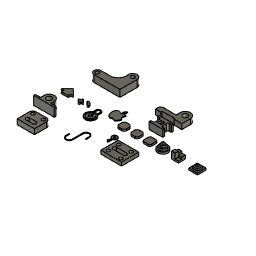
4~10 v4 (Autodesk Fusion 360 design; units mm, degrees)
Autodesk Fusion 360 part; units mm, degrees
note: some values were not read from the file. Set by a fixed rule: which sketch regions a step uses.
sketch "스케치1" plane through (0, 0, 0) normal (0, 0, 1) x (1, 0, 0)
  line L0 (-16, 16) -> (16, 16)
  line L1 (16, 16) -> (16, -16)
  line L2 (16, -16) -> (-16, -16)
  line L3 (-16, -16) -> (-16, 16)
  line L4 (-16, 16) -> (16, -16) construction
  line L5 (16, 16) -> (-16, -16) construction
  circle A0 centre (-16, 16) radius 17
  line L6 (-13, 13) -> (13, 13)
  line L7 (13, 13) -> (13, -13)
  line L8 (13, -13) -> (-13, -13)
  line L9 (-13, -13) -> (-13, 13)
  line L10 (-13, 13) -> (13, -13) construction
  line L11 (13, 13) -> (-13, -13) construction
  circle A1 centre (-13, -13) radius 12
  arc A2 (-32.6238, 19.5565) -> (-22.3496, -20.5223) centre (16.6071, 10.8206) ccw
  circle A3 centre (13, -13) radius 12
  circle A4 centre (0, -30.7482) radius 10
  circle A5 centre (16, 16) radius 17
  circle A6 centre (0, 37.7486) radius 10
  arc A7 (23.2744, -19.1998) -> (32.5898, 19.7118) centre (-16.632, 10.9247) ccw
  circle A8 centre (40, 16) radius 18
  arc A9 (-5.9259, 29.6935) -> (5.9259, 29.6935) centre (0, 37.7486) ccw
  arc A10 (5.9091, -22.6809) -> (-5.9091, -22.6809) centre (0, -30.7482) ccw
  dimension "d1" = 32
  dimension "d2" = 32
  dimension "d3" = 34
  dimension "d4" = 26
  dimension "d5" = 26
  dimension "d6" = 24
  dimension "d7" = 50
  dimension "d9" = 24
  dimension "d14" = 20
  dimension "d15" = 34
  dimension "d16" = 20
  dimension "d17" = 50
  dimension "d18" = 36
  dimension "d19" = 24
  dimension "d20" = 32
  constraint horizontal L0
  constraint perpendicular L0 L1
  constraint parallel L0 L2
  constraint parallel L1 L3
  constraint coincident L4 origin
  constraint coincident L5 origin
  constraint coincident L0.start L3.end
  constraint horizontal L6
  constraint perpendicular L6 L7
  constraint parallel L6 L8
  constraint parallel L7 L9
  constraint coincident L10 origin
  constraint coincident L11 origin
  constraint coincident L8.end L9.start
  constraint tangent A1 A2
  constraint coincident A1 A2.end
  constraint coincident A0 A2.start
  constraint coincident L7.end L8.start
  constraint tangent A3 A4
  constraint tangent A1 A4
  constraint coincident L0.end L1.start
  constraint tangent A0 A6
  constraint tangent A5 A6
  constraint coincident A3 A7.start
  constraint coincident A5 A7.end
  constraint tangent A5 A9
  constraint tangent A0 A9
  constraint coincident A6 A9.end
  constraint coincident A5 A9.end
  constraint coincident A0 A9.start
  constraint tangent A1 A10
  constraint coincident A3 A10.start
  constraint coincident A4 A10.start
  constraint coincident A1 A10.end
  constraint coincident A4 A10.end
  measures "d1" distance of L1.end L2.end
  measures "d2" distance of L0.end L1.end
  measures "d3" diameter of A0
  measures "d4" distance of L7.end L8.end
  measures "d5" distance of L6.end L7.end
  measures "d6" diameter of A1
  measures "d7" radius of A2
  measures "d9" diameter of A3
  measures "d14" diameter of A4
  measures "d15" diameter of A5
  measures "d16" diameter of A6
  measures "d17" radius of A7
  measures "d18" diameter of A8
  measures "d19" distance of L1 A8.centre
  measures "d20" distance of L2 A8.centre
extrude "돌출1" add sketch "스케치1" along normal blind 4 contours L0 L1 A0 A5 A8 | L0 A0 L6 A5 | L0 A0 A5 | L0 L1 A0 L6 L7 A5 | L0 L3 A0 L6 L9 A5 | L0 L3 A0 A2 A5 | A0 A5 A6 A9 | A0 L6 L7 A5 | A0 L6 A5 | L1 A3 A5 A7 A8 | L1 L7 A3 A5 | A0 L6 L9 A5 | A0 L7 L8 L9 A1 A3 A5 | L1 L2 A3 | L1 L2 L7 L8 A3 | L3 A0 L9 A1 | L3 A0 A1 A2 | L7 L8 A3 | L2 L3 L8 L9 A1 | L2 L3 A1 | L8 L9 A1 | L2 A1 A3 A4 A10 | L2 L8 A1 A3 makes body 1
sketch "스케치2" plane through (0, 0, 0) normal (0, 0, 1) x (1, 0, 0)
  arc A0 (-5.9259, 29.6935) -> (-32.6238, 19.5565) centre (-16, 16) ccw
  arc A1 (27.2708, 28.7267) -> (5.9259, 29.6935) centre (16, 16) ccw
  arc A2 (-5.9259, 29.6935) -> (5.9259, 29.6935) centre (0, 37.7486) ccw
  arc A3 (0, 33.006) -> (12.0073, 53.7864) centre (-6.1442, 50.4155) ccw
  arc A4 (12.0073, 53.7864) -> (0, 33.006) centre (21.5511, 34.4126) ccw
  line L0 (-16, 33) -> (16, 33)
  dimension "d24" = 24
  dimension "d35" = 16
  constraint coincident A0 L0.start
  constraint coincident A1 L0.end
  constraint tangent A1 L0
  constraint horizontal L0
  measures "d24" distance of A3.end A3.start
  measures "d35" horizontal distance of A3.start L0.start
extrude "돌출2" add sketch "스케치2" along normal blind 4 separate body contours A3 A4 makes body 2
move_body "이동1" bodies 1 2 to x (1, 0, 0) y (0, 0, 1) z (0, -1, 0) at (0, 37.7486, 22.2514)
sketch "스케치3" plane through (0, 0, 0) normal (0, 0, 1) x (1, 0, 0)
  line L0 (67.5, 22.5) -> (82.5, 22.5)
  line L1 (97.5, 7.5) -> (97.5, -7.5)
  line L2 (82.5, -22.5) -> (67.5, -22.5)
  line L3 (52.5, -7.5) -> (52.5, 7.5)
  line L4 (52.5, 22.5) -> (97.5, -22.5) construction
  line L5 (97.5, 22.5) -> (52.5, -22.5) construction
  arc A0 (67.5, 22.5) -> (52.5, 7.5) centre (67.5, 7.5) ccw
  arc A1 (97.5, 7.5) -> (82.5, 22.5) centre (82.5, 7.5) ccw
  arc A2 (52.5, -7.5) -> (67.5, -22.5) centre (67.5, -7.5) ccw
  arc A3 (82.5, -22.5) -> (97.5, -7.5) centre (82.5, -7.5) ccw
  line L6 (137.5, 22.5) -> (162.5, 22.5)
  line L7 (172.5, 12.5) -> (172.5, -12.5)
  line L8 (162.5, -22.5) -> (137.5, -22.5)
  line L9 (127.5, -12.5) -> (127.5, 12.5)
  line L10 (127.5, 22.5) -> (172.5, -22.5) construction
  line L11 (172.5, 22.5) -> (127.5, -22.5) construction
  line L12 (137.5, 22.5) -> (127.5, 12.5)
  line L13 (162.5, 22.5) -> (172.5, 12.5)
  line L14 (127.5, -12.5) -> (137.5, -22.5)
  line L15 (172.5, -12.5) -> (162.5, -22.5)
  line L16 (207.5, 22.5) -> (237.5, 22.5)
  line L17 (247.5, 17.5) -> (247.5, -12.5)
  line L18 (242.5, -22.5) -> (212.5, -22.5)
  line L19 (202.5, -17.5) -> (202.5, 12.5)
  line L20 (202.5, 22.5) -> (247.5, -22.5) construction
  line L21 (247.5, 22.5) -> (202.5, -22.5) construction
  line L22 (207.5, 22.5) -> (202.5, 12.5)
  line L23 (237.5, 22.5) -> (247.5, 17.5)
  line L24 (202.5, -17.5) -> (212.5, -22.5)
  line L25 (247.5, -12.5) -> (242.5, -22.5)
  point P0 (75, 0)
  point P1 (150, 0)
  point P2 (225, 0)
  dimension "d38" = 45
  dimension "d39" = 45
  dimension "d40" = 15
  dimension "d41" = 15
  dimension "d42" = 15
  dimension "d43" = 15
  dimension "d44" = 45
  dimension "d45" = 45
  dimension "d46" = 10
  dimension "d47" = 10
  dimension "d48" = 10
  dimension "d49" = 10
  dimension "d50" = 10
  dimension "d51" = 10
  dimension "d52" = 10
  dimension "d53" = 10
  dimension "d54" = 45
  dimension "d55" = 45
  dimension "d56" = 5
  dimension "d57" = 10
  dimension "d58" = 10
  dimension "d59" = 5
  dimension "d60" = 5
  dimension "d61" = 10
  dimension "d62" = 10
  dimension "d63" = 5
  constraint horizontal L0
  constraint perpendicular L0 L1
  constraint parallel L0 L2
  constraint parallel L1 L3
  constraint coincident L4 P0
  constraint coincident L5 P0
  constraint coincident L4.start L0
  constraint coincident L4.start L3
  constraint tangent L0 A0
  constraint tangent L3 A0
  constraint coincident L5.start L0
  constraint coincident L5.start L1
  constraint tangent L0 A1
  constraint tangent L1 A1
  constraint coincident L5.end L3
  constraint coincident L5.end L2
  constraint tangent L3 A2
  constraint tangent L2 A2
  constraint coincident L4.end L1
  constraint coincident L4.end L2
  constraint tangent L1 A3
  constraint tangent L2 A3
  constraint horizontal L6
  constraint perpendicular L6 L7
  constraint parallel L6 L8
  constraint parallel L7 L9
  constraint coincident L10 P1
  constraint coincident L11 P1
  constraint coincident L10.start L6
  constraint coincident L10.start L9
  constraint coincident L11.start L6
  constraint coincident L11.start L7
  constraint coincident L11.end L9
  constraint coincident L11.end L8
  constraint coincident L10.end L7
  constraint coincident L10.end L8
  constraint horizontal L16
  constraint perpendicular L16 L17
  constraint parallel L16 L18
  constraint parallel L17 L19
  constraint coincident L20 P2
  constraint coincident L21 P2
  constraint coincident L20.start L16
  constraint coincident L20.start L19
  constraint coincident L21.start L16
  constraint coincident L21.start L17
  constraint coincident L21.end L19
  constraint coincident L21.end L18
  constraint coincident L20.end L17
  constraint coincident L20.end L18
  measures "d38" distance of L4.end L5.end
  measures "d39" distance of L5.start L4.end
  measures "d40" radius of A0
  measures "d41" radius of A1
  measures "d42" radius of A2
  measures "d43" radius of A3
  measures "d44" distance of L10.end L11.end
  measures "d45" distance of L11.start L10.end
  measures "d46" distance of L10.start L6.start
  measures "d47" distance of L10.start L9.end
  measures "d48" distance of L11.start L6.end
  measures "d49" distance of L11.start L7.start
  measures "d50" distance of L11.end L9.start
  measures "d51" distance of L11.end L8.end
  measures "d52" distance of L10.end L7.end
  measures "d53" distance of L10.end L8.start
  measures "d54" distance of L20.end L21.end
  measures "d55" distance of L21.start L20.end
  measures "d56" distance of L20.start L16.start
  measures "d57" distance of L20.start L19.end
  measures "d58" distance of L21.start L16.end
  measures "d59" distance of L21.start L17.start
  measures "d60" distance of L21.end L19.start
  measures "d61" distance of L21.end L18.end
  measures "d62" distance of L20.end L17.end
  measures "d63" distance of L20.end L18.start
extrude "돌출3" add sketch "스케치3" along normal blind 10 separate body makes body 3 at (67.5, 2.5, 0) makes body 4 at (145.8333, 0.8333, 0) makes body 5 at (217.5, 4.1667, 0)
move_body "이동2" bodies 1 2 to x (1, 0, 0) y (0, 0, -1) z (0, 1, 0) at (0, 7.3096, 40.1875)
sketch "스케치4" plane through (0, 0, 0) normal (0, 0, 1) x (1, 0, 0)
  arc A0 (-140, -0.0033) -> (-150.0007, 9.99) centre (-150, -0.01) ccw
  arc A1 (-140, -0.0033) -> (-130, 0.0033) centre (-135, 0) ccw
  arc A2 (-130, 0.0033) -> (-150.0013, 19.99) centre (-150, -0.01) ccw
  arc A3 (-150.0013, 19.99) -> (-150.0007, 9.99) centre (-150.001, 14.99) ccw
  arc A4 (-135, 0) -> (-150.001, 14.99) centre (-150, -0.01) ccw construction
  line L0 (-181.1396, 10.4396) -> (-181.1396, -9.5604)
  arc A5 (-181.1396, -9.5604) -> (-171.1396, -9.5604) centre (-176.1396, -9.5604) ccw
  line L1 (-171.1396, -9.5604) -> (-171.1396, 10.4396)
  arc A6 (-171.1396, 10.4396) -> (-181.1396, 10.4396) centre (-176.1396, 10.4396) ccw
  line L2 (-176.1396, 10.4396) -> (-176.1396, -9.5604) construction
  line L3 (-186.1396, -4.5604) -> (-166.1396, -4.5604)
  arc A7 (-166.1396, -4.5604) -> (-166.1396, 5.4396) centre (-166.1396, 0.4396) ccw
  line L4 (-166.1396, 5.4396) -> (-186.1396, 5.4396)
  arc A8 (-186.1396, 5.4396) -> (-186.1396, -4.5604) centre (-186.1396, 0.4396) ccw
  line L5 (-186.1396, 0.4396) -> (-166.1396, 0.4396) construction
  line L6 (-258.7146, 39.3952) -> (-293.7146, 4.3952)
  line L7 (-293.7146, 4.3952) -> (-278.7146, 4.3952)
  line L8 (-278.7146, 4.3952) -> (-278.7146, -10.6048)
  line L9 (-278.7146, -10.6048) -> (-238.7146, -10.6048)
  line L10 (-238.7146, -10.6048) -> (-238.7146, 4.3952)
  line L11 (-238.7146, 4.3952) -> (-223.7146, 4.3952)
  line L12 (-223.7146, 4.3952) -> (-258.7146, 39.3952)
  point P0 (-176.1396, 0.4396)
  point P1 (-176.1396, 0.4396)
  dimension "d66" = 15
  dimension "d67" = 5
  dimension "d68" = 10
  dimension "d69" = 20
  dimension "d70" = 20
  dimension "d71" = 10
  dimension "d74" = 15
  dimension "d75" = 15
  dimension "d76" = 15
  dimension "d77" = 15
  dimension "d78" = 40
  constraint tangent A0 A1
  constraint tangent A1 A2
  constraint tangent A2 A3
  constraint tangent A0 A3
  constraint tangent L0 A5
  constraint tangent A5 L1
  constraint parallel L0 L1
  constraint tangent L1 A6
  constraint tangent L0 A6
  constraint vertical L2
  constraint midpoint L2 P1
  constraint tangent L3 A7
  constraint tangent A7 L4
  constraint parallel L3 L4
  constraint tangent L4 A8
  constraint tangent L3 A8
  constraint horizontal L5
  constraint midpoint L5 P1
  constraint horizontal L7
  constraint perpendicular L7 L8
  constraint perpendicular L8 L9
  constraint perpendicular L9 L10
  constraint perpendicular L8 L11
  constraint perpendicular L6 L12
  constraint equal L6 L12
  measures "d66" radius of A4
  measures "d67" radius of A1
  measures "d68" diameter of A5
  measures "d69" distance of A6.centre A5.centre
  measures "d70" distance of A8.centre A7.centre
  measures "d71" diameter of A7
  measures "d74" distance of L6.end L7.end
  measures "d75" distance of L10.end L11.end
  measures "d76" distance of L9.end L10.end
  measures "d77" distance of L7.end L8.end
  measures "d78" distance of L8.end L9.end
extrude "돌출4" add sketch "스케치4" along normal blind 10 separate body makes body 6 at (-177.8063, 2.1063, 0) makes body 7 at (-151.663, 14.8653, 0) makes body 8 at (-258.7146, 16.0619, 0)
sketch "스케치5" plane through (0, 0, 0) normal (0, 0, 1) x (1, 0, 0)
  circle A0 centre (-73.3666, -46.6567) radius 30
  circle A1 centre (-73.3666, -46.6567) radius 10
  line L0 (-75.8666, -31.6567) -> (-70.8666, -31.6567)
  line L1 (-70.8666, -31.6567) -> (-70.8666, -41.6567)
  line L2 (-70.8666, -41.6567) -> (-75.8666, -41.6567)
  line L3 (-75.8666, -41.6567) -> (-75.8666, -31.6567)
  line L4 (-75.8666, -31.6567) -> (-70.8666, -41.6567) construction
  line L5 (-70.8666, -31.6567) -> (-75.8666, -41.6567) construction
  line L6 (-73.3666, -46.6567) -> (-73.3666, -26.6567)
  point P0 (-73.3666, -36.6567)
  dimension "d81" = 60
  dimension "d82" = 20
  dimension "d85" = 15
  dimension "d86" = 5
  constraint concentric A0 A1
  constraint horizontal L0
  constraint perpendicular L0 L1
  constraint parallel L0 L2
  constraint parallel L1 L3
  constraint coincident L4 P0
  constraint coincident L5 P0
  constraint coincident A1 P0
  constraint coincident A0.centre A1.centre
  constraint vertical L6
  constraint midpoint P0 L6
  measures "d81" diameter of A0
  measures "d82" diameter of A1
  measures "d85" distance of A0.centre L0
  measures "d86" distance of L0.start L0.end
extrude "돌출5" add sketch "스케치5" along normal blind 2.5 and the other way blind 2.5 separate body makes body 9
sketch "스케치6" plane through (0, 0, 0) normal (0, 0, 1) x (1, 0, 0)
  circle A0 centre (-73.3666, -46.6567) radius 30
  circle A1 centre (-73.3666, -46.6567) radius 30
  line L0 (-88.3666, -20.6759) -> (-88.3666, -1.6567)
  arc A2 (-58.3666, -1.6567) -> (-88.3666, -1.6567) centre (-73.3666, -1.6567) ccw
  line L1 (-58.3666, -1.6567) -> (-58.3666, -20.6759)
  line L2 (-83.3666, -18.3724) -> (-83.3666, -1.6567)
  arc A3 (-63.3666, -1.6567) -> (-83.3666, -1.6567) centre (-73.3666, -1.6567) ccw
  line L3 (-63.3666, -1.6567) -> (-63.3666, -18.3724)
  dimension "d94" = 45
  dimension "d95" = 15
  dimension "d96" = 10
  constraint coincident A0 L0.start
  constraint coincident A1 L0.start
  constraint vertical L0
  constraint tangent L0 A2
  constraint coincident A0 L1.end
  constraint equal L0 L1
  constraint parallel L0 L1
  constraint coincident A0 L2.start
  constraint tangent L2 A3
  constraint coincident A1 L3.end
  constraint equal L2 L3
  constraint parallel L2 L3
  constraint concentric A2 A3
  constraint parallel L0 L2
  measures "d94" vertical distance of A0.centre A2.centre
  measures "d95" radius of A2
  measures "d96" radius of A3
extrude "돌출6" add sketch "스케치6" along normal blind 1.5 and the other way blind 1.5 contours A0 A1 L0 A2 L1 L2 A3 L3 bodies 9
sketch "스케치7" plane through (0, 0, 2.5) normal (0, 0, 1) x (-1, 0, 0)
  line L0 (75.8666, 36.9742) -> (75.8666, 31.6567)
  line L1 (75.8666, 31.6567) -> (70.8666, 31.6567)
  line L2 (70.8666, 31.6567) -> (70.8666, 36.9742)
  arc A0 (75.8666, 36.9742) -> (70.8666, 36.9742) centre (73.3666, 46.6567) ccw
  circle A1 centre (73.3666, 46.6567) radius 30
  circle A2 centre (73.3666, 46.6567) radius 22.5
  line L3 (75.8666, 31.6567) -> (75.8666, 36.9742)
  dimension "d101" = 45
  constraint concentric A0 A2
  constraint coincident L0.end L1.start
  constraint coincident L0.start A0.start
  measures "d101" diameter of A2
extrude "돌출7" add sketch "스케치7" along normal blind 1.5 contours A2 bodies 9
sketch "스케치8" plane through (0, 0, -2.5) normal (0, 0, -1) x (1, 0, 0)
  line L0 (-75.8666, 31.6567) -> (-75.8666, 36.9742)
  arc A0 (-70.8666, 36.9742) -> (-75.8666, 36.9742) centre (-73.3666, 46.6567) ccw
  line L1 (-70.8666, 36.9742) -> (-70.8666, 31.6567)
  line L2 (-70.8666, 31.6567) -> (-75.8666, 31.6567)
  circle A1 centre (-73.3666, 46.6567) radius 30
  circle A2 centre (-73.3666, 46.6567) radius 22.5
  dimension "d104" = 45
  constraint concentric A0 A2
  measures "d104" diameter of A2
extrude "돌출8" add sketch "스케치8" along normal blind 1.5 contours A2 bodies 9
move_body "이동3" bodies 9 to x (1, 0, 0) y (0, 1, 0) z (0, 0, 1) at (0, 0, 7)
sketch "스케치9" plane through (0, 0, 0) normal (0, 0, 1) x (1, 0, 0)
  circle A0 centre (98, -78.3901) radius 15
  line L0 (95, -93.087) -> (95, -103.3901)
  line L1 (95, -103.3901) -> (92, -103.3901)
  line L2 (92, -103.3901) -> (92, -106.3901)
  line L3 (92, -106.3901) -> (95, -106.3901)
  line L4 (95, -106.3901) -> (95, -109.3901)
  line L5 (95, -109.3901) -> (89, -109.3901)
  line L6 (89, -109.3901) -> (89, -112.3901)
  line L7 (89, -112.3901) -> (95, -112.3901)
  line L8 (95, -112.3901) -> (95, -118.3901)
  arc A1 (95, -118.3901) -> (101, -118.3901) centre (98, -118.3901) ccw
  line L9 (101, -118.3901) -> (101, -93.087)
  line L10 (98, -78.3901) -> (98, -181.0972)
  circle A2 centre (98, -78.3901) radius 6
  dimension "d107" = 30
  dimension "d108" = 40
  dimension "d109" = 6
  dimension "d110" = 3
  dimension "d111" = 3
  dimension "d112" = 3
  dimension "d113" = 6
  dimension "d114" = 3
  dimension "d116" = 6
  dimension "d117" = 6
  dimension "d118" = 3
  dimension "d119" = 12
  constraint coincident A0 L0.start
  constraint vertical L0
  constraint perpendicular L0 L1
  constraint perpendicular L1 L2
  constraint perpendicular L2 L3
  constraint perpendicular L1 L4
  constraint perpendicular L4 L5
  constraint perpendicular L5 L6
  constraint perpendicular L6 L7
  constraint perpendicular L5 L8
  constraint tangent L8 A1
  constraint coincident A0 L9.end
  constraint tangent A1 L9
  constraint parallel L8 L9
  constraint coincident A0.centre L10.start
  constraint parallel L0 L10
  constraint coincident A1.centre L10
  constraint concentric A0 A2
  measures "d107" diameter of A0
  measures "d108" distance of A0.centre A1.centre
  measures "d109" distance of L7.end L8.end
  measures "d110" distance of L5.end L6.end
  measures "d111" distance of L3.end L4.end
  measures "d112" distance of L1.end L2.end
  measures "d113" distance of L6.end L7.end
  measures "d114" radius of A1
  measures "d116" distance of L4 L9
  measures "d117" distance of L0 L9
  measures "d118" distance of L0.end L1.end
  measures "d119" diameter of A2
extrude "돌출9" add sketch "스케치9" along normal blind 3 separate body makes body 10
sketch "스케치10" plane through (0, 0, 0) normal (0, 0, 1) x (1, 0, 0)
  line L0 (21, -170) -> (21, -150)
  arc A0 (21, -150) -> (-13, -150) centre (4, -150) ccw
  line L1 (-13, -150) -> (-13, -210)
  arc A1 (-53, -210) -> (-13, -210) centre (-33, -210) ccw
  line L2 (-53, -210) -> (-53, -190)
  line L3 (-53, -190) -> (-50, -190)
  line L4 (-50, -190) -> (-50, -210)
  arc A2 (-50, -210) -> (-16, -210) centre (-33, -210) ccw
  line L5 (-16, -210) -> (-16, -150)
  arc A3 (24, -150) -> (-16, -150) centre (4, -150) ccw
  line L6 (24, -150) -> (24, -170)
  line L7 (24, -170) -> (21, -170)
  dimension "d122" = 20
  dimension "d123" = 20
  dimension "d124" = 17
  dimension "d125" = 20
  dimension "d126" = 60
  dimension "d127" = 60
  dimension "d128" = 17
  dimension "d129" = 20
  dimension "d130" = 20
  constraint vertical L0
  constraint tangent L0 A0
  constraint parallel L0 L1
  constraint tangent L1 A1
  constraint tangent A1 L2
  constraint parallel L0 L2
  constraint perpendicular L2 L3
  constraint perpendicular L3 L4
  constraint tangent L4 A2
  constraint tangent A2 L5
  constraint perpendicular L3 L5
  constraint tangent L5 A3
  constraint tangent A3 L6
  constraint perpendicular L3 L6
  constraint perpendicular L6 L7
  constraint concentric A0 A3
  constraint concentric A1 A2
  measures "d122" distance of A3.start L6.end
  measures "d123" distance of L0.start L0.end
  measures "d124" radius of A0
  measures "d125" radius of A3
  measures "d126" distance of A0.end L1.end
  measures "d127" distance of A2.end L5.end
  measures "d128" radius of A2
  measures "d129" radius of A1
  measures "d130" distance of A1.start L2.end
extrude "돌출10" add sketch "스케치10" along normal blind 3 separate body makes body 11
sketch "스케치11" plane through (0, 0, 0) normal (0, 0, 1) x (1, 0, 0)
  line L0 (-300, -150) -> (-300, -140)
  line L1 (-300, -140) -> (-270, -140)
  line L2 (-270, -140) -> (-270, -120)
  arc A0 (-210, -120) -> (-270, -120) centre (-240, -120) ccw
  line L3 (-210, -120) -> (-210, -140)
  line L4 (-210, -140) -> (-180, -140)
  line L5 (-180, -140) -> (-180, -150)
  line L6 (-180, -150) -> (-300, -150)
  circle A1 centre (-240, -120) radius 15
  dimension "d133" = 120
  dimension "d136" = 10
  dimension "d139" = 30
  dimension "d140" = 30
  constraint vertical L0
  constraint perpendicular L0 L1
  constraint perpendicular L1 L2
  constraint tangent L2 A0
  constraint tangent A0 L3
  constraint perpendicular L1 L3
  constraint perpendicular L2 L4
  constraint perpendicular L4 L5
  constraint perpendicular L0 L6
  constraint concentric A0 A1
  measures "d133" distance of L0.start L5.end
  measures "d136" distance of L0.start L0.end
  measures "d139" radius of A0
  measures "d140" diameter of A1
extrude "돌출11" add sketch "스케치11" along normal blind 50 separate body makes body 12
sketch "스케치12" plane through (0, 0, 0) normal (0, 0, 1) x (1, 0, 0)
  line L0 (140, -100) -> (260, -100)
  line L1 (260, -100) -> (260, -200)
  line L2 (260, -200) -> (140, -200)
  line L3 (140, -200) -> (140, -100)
  line L4 (140, -100) -> (260, -200) construction
  line L5 (260, -100) -> (140, -200) construction
  line L6 (170, -160) -> (230, -160)
  arc A0 (230, -160) -> (230, -140) centre (230, -150) ccw
  line L7 (230, -140) -> (170, -140)
  arc A1 (170, -140) -> (170, -160) centre (170, -150) ccw
  line L8 (170, -150) -> (230, -150) construction
  circle A2 centre (164, -120) radius 10
  circle A3 centre (164, -180) radius 10
  circle A4 centre (236, -120) radius 10
  circle A5 centre (240, -183.3333) radius 10
  point P0 (200, -150)
  point P1 (200, -150)
  dimension "d143" = 120
  dimension "d144" = 100
  dimension "d146" = 10
  dimension "d147" = 20
  dimension "d148" = 20
  dimension "d149" = 60
  dimension "d150" = 20
  dimension "d151" = 20
  dimension "d152" = 20
  dimension "d153" = 20
  dimension "d154" = 20
  dimension "d155" = 20
  constraint horizontal L0
  constraint perpendicular L0 L1
  constraint parallel L0 L2
  constraint parallel L1 L3
  constraint coincident L4 P1
  constraint coincident L5 P1
  constraint tangent L6 A0
  constraint tangent A0 L7
  constraint parallel L6 L7
  constraint tangent L7 A1
  constraint tangent L6 A1
  constraint horizontal L8
  constraint midpoint L8 P1
  constraint midpoint L4 P1
  constraint coincident L4 A2.centre
  constraint coincident L5 A3.centre
  constraint coincident L5 A4.centre
  constraint coincident L4 A5.centre
  measures "d143" distance of L1.end L2.end
  measures "d144" distance of L0.end L1.end
  measures "d146" radius of A0
  measures "d147" diameter of A2
  measures "d148" distance of L0 A2.centre
  measures "d149" distance of A1.centre A0.centre
  measures "d150" diameter of A3
  measures "d151" distance of L2 A3.centre
  measures "d152" diameter of A4
  measures "d153" distance of L0 A4.centre
  measures "d154" diameter of A5
  measures "d155" distance of L1 A5.centre
extrude "돌출12" add sketch "스케치12" along normal blind 20 separate body makes body 13
sketch "스케치13" plane through (0, 0, 0) normal (0, 0, 1) x (1, 0, 0)
  line L0 (155.8924, 123.8135) -> (235.8924, 123.8135)
  line L1 (235.8924, 123.8135) -> (235.8924, 113.8135)
  line L2 (235.8924, 113.8135) -> (225.8924, 113.8135)
  arc A0 (225.8924, 113.8135) -> (215.8924, 103.8135) centre (225.8924, 103.8135) ccw
  line L3 (215.8924, 103.8135) -> (215.8924, 83.8135)
  arc A1 (215.8924, 83.8135) -> (225.8924, 73.8135) centre (225.8924, 83.8135) ccw
  line L4 (225.8924, 73.8135) -> (235.8924, 73.8135)
  line L5 (235.8924, 73.8135) -> (235.8924, 63.8135)
  line L6 (235.8924, 63.8135) -> (155.8924, 63.8135)
  line L7 (155.8924, 63.8135) -> (155.8924, 73.8135)
  line L8 (155.8924, 73.8135) -> (165.8924, 73.8135)
  arc A2 (165.8924, 73.8135) -> (175.8924, 83.8135) centre (165.8924, 83.8135) ccw
  line L9 (175.8924, 83.8135) -> (175.8924, 103.8135)
  arc A3 (175.8924, 103.8135) -> (165.8924, 113.8135) centre (165.8924, 103.8135) ccw
  line L10 (165.8924, 113.8135) -> (155.8924, 113.8135)
  line L11 (155.8924, 113.8135) -> (155.8924, 123.8135)
  line L12 (185.8924, 103.8135) -> (205.8924, 103.8135)
  line L13 (205.8924, 103.8135) -> (205.8924, 83.8135)
  line L14 (205.8924, 83.8135) -> (185.8924, 83.8135)
  line L15 (185.8924, 83.8135) -> (185.8924, 103.8135)
  line L16 (185.8924, 103.8135) -> (205.8924, 83.8135) construction
  line L17 (205.8924, 103.8135) -> (185.8924, 83.8135) construction
  point P0 (195.8924, 93.8135)
  dimension "d158" = 80
  dimension "d159" = 10
  dimension "d160" = 10
  dimension "d161" = 10
  dimension "d162" = 10
  dimension "d164" = 40
  dimension "d166" = 20
  dimension "d167" = 10
  dimension "d168" = 10
  dimension "d169" = 20
  dimension "d170" = 10
  dimension "d171" = 10
  dimension "d172" = 40
  dimension "d173" = 20
  dimension "d174" = 20
  dimension "d175" = 20
  dimension "d176" = 10
  constraint horizontal L0
  constraint perpendicular L0 L1
  constraint perpendicular L1 L2
  constraint tangent L2 A0
  constraint tangent A0 L3
  constraint perpendicular L2 L3
  constraint tangent L3 A1
  constraint tangent A1 L4
  constraint perpendicular L1 L4
  constraint perpendicular L2 L5
  constraint perpendicular L5 L6
  constraint perpendicular L6 L7
  constraint perpendicular L7 L8
  constraint tangent L8 A2
  constraint tangent A2 L9
  constraint perpendicular L6 L9
  constraint tangent L9 A3
  constraint tangent A3 L10
  constraint perpendicular L9 L10
  constraint perpendicular L0 L11
  constraint equal L0 L6
  constraint horizontal L12
  constraint perpendicular L12 L13
  constraint parallel L12 L14
  constraint parallel L13 L15
  constraint coincident L16 P0
  constraint coincident L17 P0
  measures "d158" distance of L5.end L6.end
  measures "d159" distance of L6.end L7.end
  measures "d160" distance of L4.end L5.end
  measures "d161" distance of L0.end L1.end
  measures "d162" distance of L0.start L10.end
  measures "d164" distance of L3 L9
  measures "d166" distance of L3 L5
  measures "d167" radius of A2
  measures "d168" radius of A1
  measures "d169" distance of L9 L11
  measures "d170" radius of A3
  measures "d171" radius of A0
  measures "d172" distance of L8 L10
  measures "d173" distance of L13.end L14.end
  measures "d174" distance of L12.end L13.end
  measures "d175" distance of L0 L12
  measures "d176" distance of L3 L13
extrude "돌출13" add sketch "스케치13" along normal blind 40 separate body makes body 14
sketch "스케치14" plane through (0, 0, 0) normal (0, 0, 1) x (1, 0, 0)
  line L0 (-230, -205) -> (-170, -205)
  line L1 (-150, -225) -> (-150, -295)
  line L2 (-150, -295) -> (-250, -295)
  line L3 (-250, -295) -> (-250, -225)
  line L4 (-250, -205) -> (-150, -295) construction
  line L5 (-150, -205) -> (-250, -295) construction
  arc A0 (-230, -205) -> (-250, -225) centre (-230, -225) ccw
  arc A1 (-150, -225) -> (-170, -205) centre (-170, -225) ccw
  line L6 (-220, -275) -> (-180, -275)
  arc A2 (-180, -275) -> (-180, -255) centre (-180, -265) ccw
  line L7 (-180, -255) -> (-220, -255)
  arc A3 (-220, -255) -> (-220, -275) centre (-220, -265) ccw
  line L8 (-220, -265) -> (-180, -265) construction
  circle A4 centre (-230, -223) radius 10
  circle A5 centre (-170, -223) radius 10
  point P0 (-200, -250)
  dimension "d179" = 100
  dimension "d180" = 90
  dimension "d181" = 20
  dimension "d182" = 20
  dimension "d183" = 20
  dimension "d185" = 30
  dimension "d186" = 40
  dimension "d187" = 30
  dimension "d188" = 20
  dimension "d189" = 20
  dimension "d190" = 20
  dimension "d191" = 20
  constraint horizontal L0
  constraint perpendicular L0 L1
  constraint parallel L0 L2
  constraint parallel L1 L3
  constraint coincident L4 P0
  constraint coincident L5 P0
  constraint coincident L4.start L0
  constraint coincident L4.start L3
  constraint tangent L0 A0
  constraint tangent L3 A0
  constraint coincident L5.start L0
  constraint coincident L5.start L1
  constraint tangent L0 A1
  constraint tangent L1 A1
  constraint tangent L6 A2
  constraint tangent A2 L7
  constraint parallel L6 L7
  constraint tangent L7 A3
  constraint tangent L6 A3
  constraint parallel L2 L8
  constraint coincident L4 A4.centre
  constraint coincident L5 A5.centre
  measures "d179" distance of L1.end L2.end
  measures "d180" distance of L5.start L1.end
  measures "d181" radius of A0
  measures "d182" radius of A1
  measures "d183" diameter of A2
  measures "d185" distance of L2 A2.centre
  measures "d186" distance of A3.centre A2.centre
  measures "d187" distance of L3 A3.centre
  measures "d188" diameter of A4
  measures "d189" diameter of A5
  measures "d190" distance of L1 A5.centre
  measures "d191" distance of L3 A4.centre
extrude "돌출14" add sketch "스케치14" along normal blind 30 separate body makes body 15
sketch "스케치15" plane through (0, 0, 0) normal (0, 0, 1) x (1, 0, 0)
  line L0 (-89.6849, 140) -> (-89.6849, 240)
  arc A0 (-180, 180) -> (-139.4046, 236.2667) centre (-188.9028, 229.201) ccw
  line L1 (-180, 180) -> (-239.6849, 180)
  arc A1 (-239.6849, 180) -> (-239.6849, 140) centre (-239.6849, 160) ccw
  line L2 (-239.6849, 140) -> (-89.6849, 140)
  arc A2 (-89.6849, 240) -> (-139.4046, 236.2667) centre (-114.6849, 240) ccw
  circle A3 centre (-239.6849, 160) radius 10
  circle A4 centre (-114.6849, 240) radius 11
  dimension "d200" = 100
  dimension "d201" = 50
  dimension "d205" = 25
  dimension "d207" = 40
  dimension "d208" = 20
  dimension "d209" = 150
  dimension "d210" = 20
  dimension "d211" = 22
  constraint tangent L0 A2
  constraint parallel L1 L2
  constraint vertical L0
  constraint horizontal L2
  constraint concentric A1 A3
  constraint concentric A2 A4
  measures "d200" distance of L0.start L0.end
  measures "d201" radius of A0
  measures "d205" radius of A2
  measures "d207" distance of L1 L2
  measures "d208" radius of A1
  measures "d209" distance of L0.start A1.end
  measures "d210" diameter of A3
  measures "d211" diameter of A4
extrude "돌출15" add sketch "스케치15" along normal blind 40 separate body makes body 16
sketch "스케치16" plane through (0, 0, 0) normal (0, 0, 1) x (1, 0, 0)
  line L0 (251.7174, 158) -> (206.7174, 158)
  line L1 (206.7174, 158) -> (206.7174, 163)
  line L2 (206.7174, 163) -> (131.7174, 163)
  line L3 (131.7174, 163) -> (131.7174, 155)
  line L4 (131.7174, 155) -> (101.7174, 155)
  line L5 (101.7174, 155) -> (101.7174, 175)
  line L6 (111.7174, 185) -> (191.7174, 185)
  line L7 (191.7174, 185) -> (191.7174, 208)
  arc A0 (251.7174, 208) -> (191.7174, 208) centre (221.7174, 208) ccw
  line L8 (251.7174, 208) -> (251.7174, 158)
  line L9 (111.7174, 185) -> (101.7174, 175)
  circle A1 centre (221.7174, 208) radius 15
  point P0 (101.7174, 185)
  dimension "d214" = 45
  dimension "d215" = 90
  dimension "d216" = 5
  dimension "d217" = 30
  dimension "d218" = 50
  dimension "d220" = 8
  dimension "d221" = 30
  dimension "d222" = 75
  dimension "d224" = 30
  dimension "d225" = 10
  dimension "d226" = 10
  dimension "d227" = 30
  constraint horizontal L0
  constraint perpendicular L0 L1
  constraint perpendicular L1 L2
  constraint perpendicular L0 L3
  constraint perpendicular L3 L4
  constraint perpendicular L4 L5
  constraint perpendicular L5 L6
  constraint perpendicular L4 L7
  constraint tangent L7 A0
  constraint tangent A0 L8
  constraint coincident P0 L6
  constraint coincident P0 L5
  constraint concentric A0 A1
  measures "d214" distance of L0.start L0.end
  measures "d215" angle of L0 L8
  measures "d216" distance of L0.end L1.end
  measures "d217" distance of L4 L6
  measures "d218" distance of L0 A0.centre
  measures "d220" distance of L2 L4
  measures "d221" distance of L3.end L4.end
  measures "d222" distance of L1.end L2.end
  measures "d224" radius of A0
  measures "d225" distance of P0 L6.start
  measures "d226" distance of P0 L5.end
  measures "d227" diameter of A1
extrude "돌출16" add sketch "스케치16" along normal blind 30 separate body makes body 17
sketch "스케치17" plane through (0, 0, 0) normal (0, 0, 1) x (1, 0, 0)
  line L0 (475, 25) -> (525, 25)
  line L1 (525, 25) -> (525, -25)
  line L2 (525, -25) -> (475, -25)
  line L3 (475, -25) -> (475, 25)
  line L4 (475, 25) -> (525, -25) construction
  line L5 (525, 25) -> (475, -25) construction
  point P0 (500, 0)
  dimension "d230" = 50
  dimension "d231" = 50
  constraint horizontal L0
  constraint perpendicular L0 L1
  constraint parallel L0 L2
  constraint parallel L1 L3
  constraint coincident L4 P0
  constraint coincident L5 P0
  measures "d230" distance of L1.end L2.end
  measures "d231" distance of L0.end L1.end
extrude "돌출17" add sketch "스케치17" along normal blind 10 separate body makes body 18
sketch "스케치18" plane through (0, 0, 10) normal (0, 0, 1) x (-1, 0, 0)
  line L0 (-475, 25) -> (-525, 25)
  line L1 (-525, 25) -> (-525, -25)
  line L2 (-525, -25) -> (-475, -25)
  line L3 (-475, -25) -> (-475, 25)
  line L4 (-475, -25) -> (-525, 25)
  line L5 (-525, -25) -> (-475, 25)
  line L6 (-485, -15) -> (-515, -15)
  line L7 (-515, -15) -> (-515, 15)
  line L8 (-515, 15) -> (-485, 15)
  line L9 (-485, 15) -> (-485, -15)
  line L10 (-485, -15) -> (-515, 15) construction
  line L11 (-515, -15) -> (-485, 15) construction
  point P0 (-500, 0)
  dimension "d234" = 30
  dimension "d235" = 30
  constraint coincident L2.end L3.start
  constraint coincident L0.end L1.start
  constraint coincident L1.end L2.start
  constraint coincident L0.start L3.end
  constraint horizontal L6
  constraint perpendicular L6 L7
  constraint parallel L6 L8
  constraint parallel L7 L9
  constraint coincident L10 P0
  constraint coincident L11 P0
  constraint midpoint L5 P0
  measures "d234" distance of L7.end L8.end
  measures "d235" distance of L6.end L7.end
extrude "돌출18" add sketch "스케치18" along normal blind 10 contours L4 L5 L9 | L4 L5 L8 | L4 L5 L7 | L4 L5 L6 bodies 18
sketch "스케치19" plane through (0, 0, 20) normal (0, 0, 1) x (-1, 0, 0)
  line L0 (-485, 15) -> (-515, 15)
  line L1 (-515, 15) -> (-515, -15)
  line L2 (-515, -15) -> (-485, -15)
  line L3 (-485, -15) -> (-485, 15)
  line L4 (-485, -15) -> (-515, 15)
  line L5 (-515, -15) -> (-485, 15)
  line L6 (-495, -5) -> (-505, -5)
  line L7 (-505, -5) -> (-505, 5)
  line L8 (-505, 5) -> (-495, 5)
  line L9 (-495, 5) -> (-495, -5)
  line L10 (-495, -5) -> (-505, 5) construction
  line L11 (-505, -5) -> (-495, 5) construction
  point P0 (-500, 0)
  dimension "d238" = 10
  dimension "d239" = 10
  constraint coincident L2.end L3.start
  constraint coincident L0.end L1.start
  constraint coincident L1.end L2.start
  constraint coincident L0.start L3.end
  constraint horizontal L6
  constraint perpendicular L6 L7
  constraint parallel L6 L8
  constraint parallel L7 L9
  constraint coincident L10 P0
  constraint coincident L11 P0
  constraint midpoint L4 P0
  measures "d238" distance of L7.end L8.end
  measures "d239" distance of L6.end L7.end
extrude "돌출19" add sketch "스케치19" along normal blind 10 contours L4 L5 L9 | L4 L5 L8 | L4 L5 L7 | L4 L5 L6 bodies 18
sketch "스케치20" plane through (0, 0, 0) normal (0, 0, 1) x (1, 0, 0)
  circle A0 centre (300, 0) radius 29
  dimension "d242" = 58
  measures "d242" diameter of A0
extrude "돌출20" add sketch "스케치20" along normal blind 10 separate body makes body 19
sketch "스케치21" plane through (0, 0, 10) normal (0, 0, 1) x (-1, 0, 0)
  circle A0 centre (-300, 0) radius 29
  circle A1 centre (-300, 0) radius 21
  dimension "d245" = 42
  constraint concentric A0 A1
  measures "d245" diameter of A1
extrude "돌출21" add sketch "스케치21" along normal blind 10 contours A1 bodies 19
sketch "스케치22" plane through (0, 0, 20) normal (0, 0, 1) x (-1, 0, 0)
  circle A0 centre (-300, 0) radius 21
  circle A1 centre (-300, 0) radius 13
  dimension "d248" = 26
  constraint concentric A0 A1
  measures "d248" diameter of A1
extrude "돌출22" add sketch "스케치22" along normal blind 10 contours A1 bodies 19
sketch "스케치23" plane through (0, 0, 30) normal (0, 0, 1) x (-1, 0, 0)
  circle A0 centre (-300, 0) radius 13
  circle A1 centre (-300, 0) radius 5
  dimension "d251" = 10
  constraint concentric A0 A1
  measures "d251" diameter of A1
extrude "돌출23" add sketch "스케치23" along normal blind 10 contours A1 bodies 19
sketch "스케치24" plane through (0, 0, 0) normal (0, 0, 1) x (1, 0, 0)
  line L0 (370, 20) -> (410, 20)
  line L1 (410, 20) -> (410, -20)
  line L2 (410, -20) -> (370, -20)
  line L3 (370, -20) -> (370, 20)
  line L4 (370, 20) -> (410, -20) construction
  line L5 (410, 20) -> (370, -20) construction
  point P0 (390, 0)
  dimension "d254" = 40
  dimension "d255" = 40
  constraint horizontal L0
  constraint perpendicular L0 L1
  constraint parallel L0 L2
  constraint parallel L1 L3
  constraint coincident L4 P0
  constraint coincident L5 P0
  measures "d254" distance of L1.end L2.end
  measures "d255" distance of L0.end L1.end
extrude "돌출24" add sketch "스케치24" along normal blind 10 separate body makes body 20
sketch "스케치25" plane through (0, 0, 10) normal (0, 0, 1) x (-1, 0, 0)
  line L0 (-370, 20) -> (-410, 20)
  line L1 (-410, 20) -> (-410, -20)
  line L2 (-410, -20) -> (-370, -20)
  line L3 (-370, -20) -> (-370, 20)
  line L4 (-410, -20) -> (-390, -20)
  line L5 (-390, -20) -> (-390, 0)
  line L6 (-390, 0) -> (-410, 0)
  line L7 (-410, 0) -> (-410, -20)
  dimension "d258" = 20
  dimension "d259" = 20
  constraint horizontal L4
  constraint vertical L5
  constraint horizontal L6
  constraint vertical L7
  constraint coincident L1.end L2.start
  measures "d258" distance of L1.end L4.end
  measures "d259" distance of L1.end L6.end
extrude "돌출25" add sketch "스케치25" along normal blind 10 contours L1 L2 L4 L5 L6 L7 bodies 20
sketch "스케치26" plane through (0, 0, 10) normal (0, 0, 1) x (-1, 0, 0)
  line L0 (-390, 0) -> (-390, -20)
  line L1 (-390, -20) -> (-370, -20)
  line L2 (-370, -20) -> (-370, 20)
  line L3 (-370, 20) -> (-410, 20)
  line L4 (-410, 20) -> (-410, 0)
  line L5 (-410, 0) -> (-390, 0)
  line L6 (-370, -20) -> (-390, -20)
  line L7 (-390, -20) -> (-390, 0)
  line L8 (-390, 0) -> (-370, 0)
  line L9 (-370, 0) -> (-370, -20)
  constraint horizontal L6
  constraint vertical L7
  constraint horizontal L8
  constraint vertical L9
  constraint coincident L0.start L5.end
  constraint coincident L1.end L2.start
extrude "돌출26" add sketch "스케치26" along normal blind 20 contours L0 L1 L2 L6 L7 L8 L9 bodies 20
sketch "스케치27" plane through (0, 0, 10) normal (0, 0, 1) x (-1, 0, 0)
  line L0 (-410, 0) -> (-370, 0)
  line L1 (-370, 0) -> (-370, 20)
  line L2 (-370, 20) -> (-410, 20)
  line L3 (-410, 20) -> (-410, 0)
  line L4 (-370, 0) -> (-390, 0)
  line L5 (-390, 0) -> (-390, 20)
  line L6 (-390, 20) -> (-370, 20)
  line L7 (-370, 20) -> (-370, 0)
  constraint horizontal L4
  constraint vertical L5
  constraint horizontal L6
  constraint vertical L7
  constraint midpoint L2 L5.end
  constraint coincident L0.end L1.start
extrude "돌출27" add sketch "스케치27" along normal blind 30 contours L0 L1 L2 L4 L5 L6 L7 bodies 20
equation "d47 = d46"
equation "d49 = d48"
equation "d51 = d50"
equation "d53 = d52"
equation "d226 = d225"
